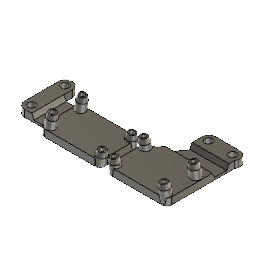
CamHolders (Autodesk Fusion 360 design; units mm, degrees)
Autodesk Fusion 360 part; units mm, degrees
sketch "Sketch1" plane through (0, 0, 0) normal (0, 0, 1) x (1, 0, 0)
  circle A0 centre (14, 15.5) radius 1.6
  circle A1 centre (24, 15.5) radius 1.6
  circle A2 centre (-36, 5.5) radius 1.6
  circle A3 centre (-36, -8.5) radius 1.6
  line L0 (-39.5, 0) -> (46.5, 0) construction
  line L1 (0, -10) -> (0, 24) construction
  line L2 (3.5, 0) -> (24.5, 0) construction
  line L3 (24.5, 0) -> (24.5, -12.5) construction
  line L4 (24.5, -12.5) -> (3.5, -12.5) construction
  line L5 (3.5, -12.5) -> (3.5, 0) construction
  line L6 (-3.5, 0) -> (-24.5, 0) construction
  line L7 (-24.5, 0) -> (-24.5, -12.5) construction
  line L8 (-24.5, -12.5) -> (-3.5, -12.5) construction
  line L9 (-3.5, -12.5) -> (-3.5, 0) construction
  line L10 (26.5, -14.5) -> (1.5, -14.5)
  line L11 (1.5, -14.5) -> (1.5, 2)
  line L12 (1.5, 2) -> (26.5, 2)
  line L13 (26.5, 2) -> (26.5, -14.5)
  line L14 (-1.5, 2) -> (-26.5, 2)
  line L15 (-26.5, 2) -> (-26.5, -14.5)
  line L16 (-26.5, -14.5) -> (-1.5, -14.5)
  line L17 (-1.5, -14.5) -> (-1.5, 2)
  line L18 (14, 12.5) -> (24, 12.5)
  arc A4 (24, 12.5) -> (24, 18.5) centre (24, 15.5) ccw
  line L19 (24, 18.5) -> (14, 18.5)
  arc A5 (14, 18.5) -> (14, 12.5) centre (14, 15.5) ccw
  line L20 (14, 15.5) -> (24, 15.5) construction
  line L21 (-39, 5.5) -> (-39, -8.5)
  arc A6 (-39, -8.5) -> (-33, -8.5) centre (-36, -8.5) ccw
  line L22 (-33, -8.5) -> (-33, 5.5)
  arc A7 (-33, 5.5) -> (-39, 5.5) centre (-36, 5.5) ccw
  line L23 (-36, 5.5) -> (-36, -8.5) construction
  line L24 (26.5, 2) -> (26.5, 13.8417)
  line L25 (11, 15.5) -> (11, 10)
  line L26 (-26.5, 2) -> (-33, 2)
  line L27 (26.5, 11.5) -> (11, 11.5)
  line L28 (26.5, 4.5) -> (6.9046, 4.5)
  line L29 (-33, -8.5) -> (-33, -11.5)
  line L30 (11, 10) -> (5.043, 2)
  line L31 (-36, -11.5) -> (-26.5, -11.5)
  dimension "d1" = 3.2
  dimension "d2" = 3.2
  dimension "d3" = 10
  dimension "d4" = 3.2
  dimension "d5" = 3.2
  dimension "d6" = 14
  dimension "d7" = 10
  dimension "d8" = 50
  dimension "d9" = 15.5
  dimension "d10" = 14
  dimension "d11" = 12.5
  dimension "d12" = 21
  dimension "d15" = 7
  dimension "d16" = 12.5
  dimension "d17" = 21
  dimension "d18" = -2
  dimension "d19" = 2
  dimension "d20" = 6
  dimension "d21" = 6
  dimension "d22" = 5.5
  dimension "d25" = 2.5
  dimension "d26" = 7
  constraint horizontal A0.centre A1.centre
  constraint horizontal L0
  constraint vertical L1
  constraint coincident origin L0
  constraint coincident origin L1
  constraint vertical A2.centre A3.centre
  constraint horizontal L2
  constraint vertical L3
  constraint horizontal L4
  constraint vertical L5
  constraint midpoint L0 L2.start
  constraint horizontal L6
  constraint vertical L7
  constraint horizontal L8
  constraint vertical L9
  constraint coincident L0 L6.start
  constraint tangent L18 A4
  constraint tangent A4 L19
  constraint parallel L18 L19
  constraint tangent L19 A5
  constraint tangent L18 A5
  constraint coincident A1.centre A4.centre
  constraint horizontal L20
  constraint coincident A0.centre A5.centre
  constraint tangent L21 A6
  constraint tangent A6 L22
  constraint parallel L21 L22
  constraint tangent L22 A7
  constraint tangent L21 A7
  constraint coincident A3.centre A6.centre
  constraint vertical L23
  constraint coincident A2.centre A7.centre
  constraint coincident A4 L24.end
  constraint perpendicular L12 L24
  constraint midpoint A5 L25.start
  constraint tangent A5 L25
  constraint vertical L25
  constraint coincident L22 L26.end
  constraint perpendicular L22 L26
  constraint coincident L24 L27.start
  constraint coincident L25 L27.end
  constraint perpendicular L25 L27
  constraint coincident L24 L28.start
  constraint perpendicular L24 L28
  constraint tangent A6 L29
  constraint coincident L12 L30.end
  constraint coincident L28.end L30
  constraint midpoint A6 L31.start
  constraint coincident L15 L31.end
  constraint tangent A6 L31
  constraint perpendicular L15 L31
  constraint coincident L29.end L31
  measures "d1" diameter of A0
  measures "d2" diameter of A1
  measures "d3" distance of A0.centre A1.centre
  measures "d4" diameter of A2
  measures "d5" diameter of A3
  measures "d6" distance of A2.centre A3.centre
  measures "d7" vertical distance of A0.centre A2.centre
  measures "d8" horizontal distance of A0.centre A2.centre
  measures "d9" distance of A1.centre L0
  measures "d10" distance of A0.centre L1
  measures "d11" distance of L2.end L3.end
  measures "d12" distance of L3.end L4.end
  measures "d15" distance of L5 L9
  measures "d16" distance of L6.end L7.end
  measures "d17" distance of L7.end L8.end
  measures "d20" diameter of A4
  measures "d21" diameter of A6
  measures "d22" distance of L25.start L25.end
  measures "d25" distance of L12 L28
  measures "d26" distance of L27 L28
extrude "Extrude1" add sketch "Sketch1" along normal blind 1 makes body 1 at (-9.8333, -8, 0) makes body 2 at (11.0143, -9, 0)
extrude "Extrude2" add sketch "Sketch1" along normal blind 3 contours L10 L11 L12 L13 | L12 L24 L28 L30 | L18 A4 A5 L24 L25 L27 | L18 A4 L19 A5 | L14 L15 L16 L17 | L21 A6 L22 A7 | A6 L29 L31 bodies 2 1
fillet "Fillet1" radius 2 8 edges at (-1.5, -14.5, 1.5) (-1.5, 2, 1.5) (-26.5, -14.5, 1.5) (1.5, -14.5, 1.5) (26.5, -14.5, 1.5) (1.5, 2, 1.5) (5.043, 2, 1.5) (11, 10, 0.5) on bodies 1 2
chamfer "Chamfer1" distance 1 distance2 2 4 edges at (-33, -4.75, 1) (-26.5, -4.75, 1) (16.7023, 4.5, 1) (18.75, 11.5, 1) measured on face at (-30.8333, -7, 1) measured on face at (-30.8333, -7, 1) measured on face at (21.3116, 8.7188, 1) measured on face at (21.3116, 8.7188, 1) on bodies 1 2
sketch "Sketch2" plane through (0, 0, 0) normal (0, 0, 1) x (1, 0, 0)
  line L0 (-24.5, 0) -> (-24.5, -12.5)
  line L1 (-3.5, -12.5) -> (-3.5, 0)
  line L2 (3.5, -12.5) -> (3.5, 0)
  line L3 (24.5, 0) -> (24.5, -12.5)
  line L4 (-3.5, 0) -> (-24.5, 0)
  line L5 (-24.5, -12.5) -> (-3.5, -12.5)
  line L6 (24.5, -12.5) -> (3.5, -12.5)
  line L7 (3.5, 0) -> (24.5, 0)
  circle A0 centre (-24.5, 0) radius 2
  circle A1 centre (-3.5, 0) radius 2
  circle A2 centre (3.5, 0) radius 2
  circle A3 centre (24.5, 0) radius 2
  circle A4 centre (24.5, -12.5) radius 2
  circle A5 centre (3.5, -12.5) radius 2
  circle A6 centre (-3.5, -12.5) radius 2
  circle A7 centre (-24.5, -12.5) radius 2
  dimension "d37" = 4
  dimension "d38" = 4
  dimension "d39" = 4
  dimension "d40" = 4
  dimension "d41" = 4
  dimension "d42" = 4
  dimension "d43" = 4
  dimension "d44" = 4
  constraint coincident L0.start L4.end
  constraint coincident L1.end L4.start
  constraint coincident L2.end L7.start
  constraint coincident L3.start L7.end
  constraint coincident L3.end L6.start
  constraint coincident L2.start L6.end
  constraint coincident L1.start L5.end
  constraint coincident L0.end L5.start
  measures "d37" diameter of A0
  measures "d38" diameter of A1
  measures "d39" diameter of A7
  measures "d40" diameter of A6
  measures "d41" diameter of A2
  measures "d42" diameter of A3
  measures "d43" diameter of A5
  measures "d44" diameter of A4
extrude "Extrude3" add sketch "Sketch2" along normal blind 1 from surface at -10 separate body contours L0 L1 L4 L5 A0 A1 A6 A7 | L2 L3 L6 L7 A2 A3 A4 A5 makes body 3 at (-16.9392, -7.9729, -10) makes body 4 at (11.0608, -7.9729, -10)
extrude "Extrude4" add sketch "Sketch2" along normal blind 18 from surface at -10 contours L0 L4 A0 | L0 L4 A0 | L0 L5 A7 | L0 L5 A7 | L1 L4 A1 | L1 L4 A1 | L1 L5 A6 | L1 L5 A6 | L2 L6 A5 | L2 L6 A5 | L2 L7 A2 | L2 L7 A2 | L3 L6 A4 | L3 L6 A4 | L3 L7 A3 | L3 L7 A3 bodies 3 4
chamfer "Chamfer2" distance 0.5 distance2 2 8 faces at (2.3225, -0.246, 8) (4.0883, -12.0466, 8) (24.1065, -12.0759, 8) (25.0109, -0.5506, 8) (-23.927, -0.4727, 8) (-24.2343, -11.5836, 8) (-3.3517, -13.15, 8) (-2.8131, 0.4683, 8) on bodies 3 4
move_body "Move1" bodies 4 to x (0.997916, 0, 0.064532) y (0, 1, 0) z (-0.064532, 0, 0.997916) at (0, 0, 0)
move_body "Move3" bodies 3 to x (0.997916, 0, -0.064532) y (0, 1, 0) z (0.064532, 0, 0.997916) at (0, 0, 0)
move_body "Move2" bodies 4 to x (1, 0, 0) y (0, 0.996195, 0.087156) z (0, -0.087156, 0.996195) at (0, 0.1271, -0.9113)
move_body "Move4" bodies 3 to x (0.996195, 0, -0.087156) y (0, 1, 0) z (0.087156, 0, 0.996195) at (-0.2089, 0, -2.7852)
combine "Combine1" operation add target body 1 tool bodies 3
combine "Combine2" operation add target body 2 tool bodies 4
hole "Hole1" at (-23.2169, 0, 8.8287) direction (-0.151261, 0, -0.988494) diameter 1.8 end through all bodies 1
hole "Hole2" at (-23.2169, -12.5, 8.8287) direction (-0.151261, 0, -0.988494) diameter 1.8 end through all bodies 1
hole "Hole3" at (-2.4586, 0, 5.6522) direction (-0.151261, 0, -0.988494) diameter 1.8 end through all bodies 1
hole "Hole4" at (-2.4586, -12.5, 5.6522) direction (-0.151261, 0, -0.988494) diameter 1.8 end through all bodies 1
hole "Hole5" at (2.9764, -0.5884, 7.2666) direction (0.064532, 0.086974, -0.994118) diameter 1.8 end through all bodies 2
hole "Hole6" at (2.9764, -13.0408, 6.1772) direction (0.064532, 0.086974, -0.994118) diameter 1.8 end through all bodies 2
hole "Hole7" at (23.9327, -0.7065, 8.6166) direction (0.064532, 0.086974, -0.994118) diameter 1.8 end through all bodies 2
hole "Hole8" at (23.9327, -13.1589, 7.5272) direction (0.064532, 0.086974, -0.994118) diameter 1.8 end through all bodies 2
split "Split1" by plane through (0, 0, 0) normal (0, 0, 1) bodies 2 1 makes body 6 at (-10.9998, -8.0488, 0) makes body 5 at (16.8767, -4.4217, 0)
delete_body "RemoveBody1" bodies 2
delete_body "RemoveBody2" bodies 1
equation "pcb_hole_dia = 1.8 mm"
equation "pcb_standoff_dia = 4 mm"
equation "pcb_standoff_dia_small = 3 mm"
equation "cam_tilt_angle = 3.7 deg"
equation "d37 = pcb_standoff_dia"
equation "d38 = d37"
equation "d39 = d37"
equation "d40 = d37"
equation "d41 = d37"
equation "d42 = d37"
equation "d43 = d37"
equation "d44 = d37"
equation "d51 = -cam_tilt_angle"
equation "cam_adjust_tilt_angle = 5 deg"
equation "d53 = cam_adjust_tilt_angle"
equation "d54 = cam_tilt_angle"
equation "d55 = cam_adjust_tilt_angle"
equation "d56 = ( pcb_standoff_dia - pcb_standoff_dia_small ) / 2"
equation "d59 = pcb_hole_dia"
equation "d62 = pcb_hole_dia"
equation "d65 = pcb_hole_dia"
equation "d68 = pcb_hole_dia"
equation "d71 = pcb_hole_dia"
equation "d74 = pcb_hole_dia"
equation "d77 = pcb_hole_dia"
equation "d80 = pcb_hole_dia"
named bodies: "CamHolderA", "CamHolderB"
